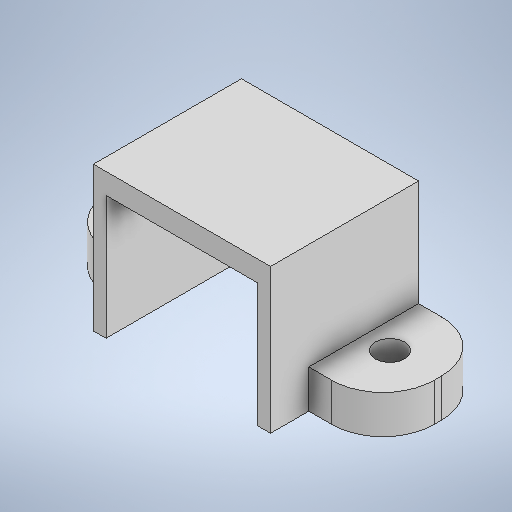
# Autodesk Inventor part: SoporteMotor_3.0
Saved by Autodesk Inventor 2025.3 (Build 293356030, 356C)
## iProperties
Created: 2025-11-04
Part Number: SoporteMotor_3.0
Material: Generic
Document SubType Name: Modeling
Designer: brene
Density: 1 g/cm^3
Appearance: Default
Author: brene
Autodesk Inventor part; units mm, degrees
ref_plane "YZ Plane" through (0, 0, 0) normal (1, 0, 0) x (0, 1, 0)
ref_plane "XZ Plane" through (0, 0, 0) normal (0, 1, 0) x (-1, 0, 0)
ref_plane "XY Plane" through (0, 0, 0) normal (0, 0, 1) x (1, 0, 0)
sketch "Sketch1" plane through (0, 0, 0) normal (0, 0, 1) x (1, 0, 0)
  line L0 (0, 0) -> (12.75, 0)
  line L1 (0, 0) -> (-12.75, 0)
  line L2 (-12.75, 0) -> (-12.75, 11.32)
  line L3 (-12.75, 11.32) -> (12.75, 11.32)
  line L4 (12.75, 11.32) -> (12.75, 0)
  line L5 (0, 0) -> (-5.95, 0)
  line L6 (0, 0) -> (5.95, 0)
  line L7 (12.75, 0) -> (6.94, 0)
  line L8 (0, 11.32) -> (0, 9.7)
  line L9 (0, 9.7) -> (6.94, 9.7)
  line L10 (6.94, 9.7) -> (6.94, 0)
  line L11 (0, 0) -> (0, 11.32)
  line L12 (0, 9.7) -> (-6.94, 9.7)
  line L13 (-6.94, 9.7) -> (-6.94, 0)
  line L14 (-12.75, 0) -> (-6.94, 0)
  line L15 (12.75, 0) -> (12.75, 3)
  line L16 (12.75, 3) -> (6.94, 3)
  line L17 (-12.75, 3) -> (-6.94, 3)
  line L18 (-6.94, 9.7) -> (-6.94, 11.32)
  line L19 (6.94, 9.7) -> (6.94, 11.32)
  line L20 (5.95, 0) -> (5.95, 9.7)
  line L21 (-5.95, 0) -> (-5.95, 9.7)
  dimension "d0" = 12.75
  dimension "d1" = 12.75
  dimension "d2" = 11.32
  dimension "d3" = 25.5
  dimension "d4" = 5.95
  dimension "d5" = 5.95
  dimension "d6" = 5.81
  dimension "d7" = 1.62
  dimension "d8" = 5.81
  dimension "d9" = 3
  constraints: 44 end point, 9 point on line, 8 perpendicular, 4 symmetric about line, 2 horizontal, 2 vertical, 1 midpoint
  measures "d0" distance of L0.start L0.end
  measures "d1" distance of L0.start L1.end
  measures "d2" distance of L1.end L2.end
  measures "d3" distance of L2.end L3.end
  measures "d4" distance of L0.start L5.end
  measures "d5" distance of L0.start L6.end
  measures "d6" distance of L0.end L7.end
  measures "d7" distance of L8.start L8.end
  measures "d8" distance of L1.end L13.end
  measures "d9" distance of L0.end L15.end
extrude "Extrusion1" add sketch "Sketch1" along normal blind 11.6 contours L20 L9 L10 L0 | L1 L13 L12 L21 | L12 L18 L3 L8 | L8 L3 L19 L9 | L10 L16 L4 L0 | L1 L2 L17 L13
sketch "Sketch2" plane through (6.94, 3, 0) normal (0, 1, 0) x (1, 0, 0)
  line L0 (-6.94, 0) -> (-6.94, -11.6)
  line L1 (-12.89, -11.6) -> (-0.99, -11.6) projected
  line L2 (-0.99, -11.6) -> (5.81, -11.6) projected
  line L3 (5.81, -11.6) -> (5.81, -8.6)
  line L4 (5.81, -8.6) -> (0, -8.6)
  line L5 (0, 0) -> (0, -11.6) projected
  line L6 (0, -11.6) -> (5.81, -11.6)
  line L7 (2.905, -8.6) -> (2.905, 0)
  line L8 (-0.99, 0) -> (5.81, 0) projected
  line L9 (5.81, 0) -> (5.81, -11.6) projected
  line L10 (5.81, -8.6) -> (5.81, 0)
  line L11 (-12.89, -11.6) -> (-19.69, -11.6)
  line L12 (-19.69, -11.6) -> (-19.69, -8.6)
  line L13 (-19.69, -8.6) -> (-13.88, -8.6)
  line L14 (-13.88, 0) -> (-13.88, -11.6)
  line L15 (-16.785, -8.6) -> (-16.785, 0)
  dimension "d12" = 3
  constraints: 22 end point, 7 symmetric about line, 3 point on line, 2 midpoint, 2 vertical, 1 collinear, 1 parallel, 1 perpendicular
  measures "d12" distance of L2.end L3.end
extrude "Extrusion2" cut sketch "Sketch2" against normal blind 11.6 contours L5 L4 L3 L2 | L11 L12 L13 L14
fillet "Fillet1" radius 4 4 edges at (-12.75, 1.5, 0) (-12.75, 1.5, 8.6) (12.75, 1.5, 0) (12.75, 1.5, 8.6)
sketch "Sketch4" plane through (6.94, 3, 8.6) normal (0, 1, 0) x (1, 0, 0)
  line L0 (5.81, 4.6) -> (5.81, 4) projected
  line L1 (5.81, 4.3) -> (-19.69, 4.3)
  line L2 (-19.69, 4.6) -> (-19.69, 4) projected
  line L3 (-6.94, 8.6) -> (-6.94, 4.3)
  line L4 (-6.94, 4.3) -> (2.06, 4.3)
  line L5 (-6.94, 4.3) -> (-15.94, 4.3)
  circle A0 centre (-15.94, 4.3) radius 1.15
  circle A1 centre (2.06, 4.3) radius 1.15
  dimension "d16" = 9
  dimension "d17" = 9
  dimension "d18" = 2.3
  dimension "d19" = 2.3
  constraints: 8 end point, 3 midpoint, 2 centre point, 2 coincident, 2 point on line
  measures "d16" distance of L3.end L4.end
  measures "d17" distance of L3.end L5.end
  measures "d18" diameter of A0
  measures "d19" diameter of A1
extrude "Extrusion3" cut sketch "Sketch4" against normal blind 11.6
body "Solid1"
